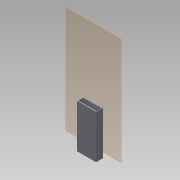
# Autodesk Inventor part: Außenhülle
Saved by Autodesk Inventor 2015 (Build 190159000, 159)
## iProperties
Created: 2016-03-24
Part Number: Außenhülle
Material: Generisch
Document SubType Name: Modeling
Designer: Bene
Density: 1 g/cm^3
Appearance: Vorgabe
Author: Bene
Autodesk Inventor part; units mm, degrees
ref_plane "YZ Plane" through (0, 0, 0) normal (1, 0, 0) x (0, 1, 0)
ref_plane "XZ Plane" through (0, 0, 0) normal (0, 1, 0) x (-1, 0, 0)
ref_plane "XY Plane" through (0, 0, 0) normal (0, 0, 1) x (1, 0, 0)
ref_plane "Arbeitsebene1" through (41.6445, -55.4632, -27.5498) normal (0, -1, 0) x (1, 0, 0)
sketch "Skizze1" plane through (41.6445, -55.4632, -27.5498) normal (0, -1, 0) x (1, 0, 0)
  line L0 (0, -17.58) -> (11, -17.58)
  line L1 (11, -17.58) -> (11, -68.08)
  line L2 (11, -68.08) -> (0, -68.08)
  line L3 (0, -68.08) -> (0, -17.58)
  line L4 (-20.1267, -68.08) -> (20.1267, -68.08) projected
  line L5 (0, 101.8556) -> (0, -98.0191)
  line L6 (0, -17.58) -> (-11, -17.58)
  line L7 (-11, -17.58) -> (-11, -68.08)
  line L8 (-11, -68.08) -> (0, -68.08)
  point P0 (-41.6445, 27.5498)
  dimension "d0" = 11
  dimension "d1" = 50.5
  constraints: 16 end point, 2 parallel, 2 symmetric about line, 1 horizontal, 1 midpoint, 1 perpendicular, 1 vertical
  measures "d0" distance of L2.end L1.end
  measures "d1" distance of L0.end L1.end
extrude "Extrusion1" add sketch "Skizze1" along normal blind 8
sketch "Skizze2" plane through (30.6445, -55.4632, -45.1298) normal (0, 0, 1) x (1, 0, 0)
  line L0 (22, 0) -> (0, 0) projected
  line L1 (0, 0) -> (0, -8) projected
  line L2 (22, -8) -> (0, -8) projected
  line L3 (22, 0) -> (22, -8) projected
  line L4 (21.5, -1.25) -> (0.5, -1.25)
  line L5 (0.5, -1.25) -> (0.5, -6.75)
  line L6 (0.5, -6.75) -> (21.5, -6.75)
  line L7 (21.5, -6.75) -> (21.5, -1.25)
  line L8 (21.5, -1.25) -> (0.5, -6.75) construction
  line L9 (0.5, -1.25) -> (21.5, -6.75) construction
  point P0 (-30.6445, 55.4632)
  point P1 (11, -4)
  dimension "d4" = 21
  dimension "d5" = 5.5
  constraints: 12 end point, 2 midpoint, 2 parallel, 1 horizontal, 1 perpendicular
  measures "d4" distance of L4.start L4.end
  measures "d5" distance of L5.end L4.end
extrude "Extrusion2" cut sketch "Skizze2" against normal blind 17.5 contours L7 L6 L5 L4
